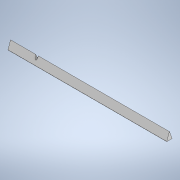
# Autodesk Inventor part: Grua Maya
Saved by Autodesk Inventor 2020 (Build 240168000, 168)
## iProperties
Created: 2019-10-05
Part Number: Grua Maya
Material: Genérico
Document SubType Name: Modeling
Designer: dasa1
Density: 1 g/cm^3
Appearance: Valor por defecto
Author: dasa1
Autodesk Inventor part; units mm, degrees
ref_plane "YZ Plane" through (0, 0, 0) normal (1, 0, 0) x (0, 1, 0)
ref_plane "XZ Plane" through (0, 0, 0) normal (0, 1, 0) x (-1, 0, 0)
ref_plane "XY Plane" through (0, 0, 0) normal (0, 0, 1) x (1, 0, 0)
sketch "Boceto1" plane through (0, 0, 0) normal (0, 1, 0) x (-1, 0, 0)
  line L0 (0, 0) -> (500, 0) construction
  line L1 (500, 0) -> (500, -50) construction
  line L2 (500, -50) -> (0, -50) construction
  line L3 (0, -50) -> (0, 0) construction
  line L4 (500, -50) -> (-2500, -50)
  line L5 (-2500, -50) -> (-2500, 50)
  line L6 (-2500, 50) -> (500, 50)
  line L7 (500, 50) -> (500, -50)
  circle A0 centre (0, 0) radius 25
  dimension "d0" = 500
  dimension "d1" = 50
  dimension "d2" = 3000
  dimension "d3" = 100
  dimension "d16" = 50
  constraints: 16 end point, 4 parallel, 2 horizontal, 2 perpendicular, 1 centre point, 1 coincident
  measures "d0" distance of L1.end L2.end
  measures "d1" distance of L0.end L1.end
  measures "d2" distance of L5.end L6.end
  measures "d3" distance of L4.end L5.end
  measures "d16" diameter of A0
extrude "Extrusión1" add sketch "Boceto1" along normal blind 140 contours L4 L5 L6 L7 | A0
chamfer "Chaflán1" distance 50 angle 70 2 edges at (1000, 140, 50) (1000, 140, -50) measured on face at (1000, 140, -49.5) measured on face at (1000, 140, 49.5)
sketch "Boceto2" plane through (0, 0, 0) normal (0, -1, 0) x (1, 0, 0)
  line L0 (-500, -50) -> (-500, 50) construction
  line L1 (-500, 50) -> (0, 50) construction
  line L2 (0, 50) -> (0, 0) construction
  line L3 (0, 0) -> (-500, 0) construction
  line L4 (-500, 0) -> (-500, 50) construction
  circle A0 centre (0, 0) radius 25
  point P0 (0, 0)
  dimension "d17" = 50
  dimension "d18" = 500
  dimension "d19" = 50
  constraints: 8 end point, 2 parallel, 1 centre point, 1 coincident, 1 horizontal, 1 perpendicular
  measures "d17" diameter of A0
  measures "d18" distance between parallel lines of L2 L0
  measures "d19" distance between parallel lines of L1 L3
hole "Agujero1" at (0, 0, 0) direction (0, 1, 0) diameter 50 end through all
